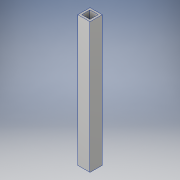
# Autodesk Inventor part: Chasis Hieght 4
Saved by Autodesk Inventor 2019.4 (Build 234330000, 330)
## iProperties
Created: 2019-01-05
Part Number: Chasis Hieght 4
Material: Aluminum 6061
Document SubType Name: Modeling
Designer: Jacob's Laptop
Density: 2.7 g/cm^3
Appearance: Aluminum - Flat
Mass: 51.8497 g
Surface Area: 125 cm^2
Volume: 19.2036 cm^3
Author: Jacob's Laptop
Autodesk Inventor part; units mm, degrees
ref_plane "YZ Plane" through (0, 0, 0) normal (1, 0, 0) x (0, 1, 0)
ref_plane "XZ Plane" through (0, 0, 0) normal (0, 1, 0) x (-1, 0, 0)
ref_plane "XY Plane" through (0, 0, 0) normal (0, 0, 1) x (1, 0, 0)
sketch "Sketch1" plane through (0, 0, 0) normal (0, 1, 0) x (-1, 0, 0)
  line L0 (0, 0) -> (-19.05, 0)
  line L1 (-19.05, 0) -> (-19.05, -19.05)
  line L2 (-19.05, -19.05) -> (0, -19.05)
  line L3 (0, -19.05) -> (0, 0)
  line L4 (-3.175, -15.875) -> (-15.875, -15.875)
  line L5 (-15.875, -15.875) -> (-15.875, -3.175)
  line L6 (-15.875, -3.175) -> (-3.175, -3.175)
  line L7 (-3.175, -3.175) -> (-3.175, -15.875)
  dimension "d0" = 19.05
  dimension "d1" = 19.05
  dimension "d2" = 3.175
  constraints: 16 end point, 4 parallel, 2 perpendicular, 1 horizontal, 3 other
  measures "d0" distance of L2.end L1.end
  measures "d1" distance of L1.end L0.end
  measures "d2" distance between parallel lines of L2 L4
extrude "Extrusion1" add sketch "Sketch1" along normal blind 203.2
body "Solid1"
